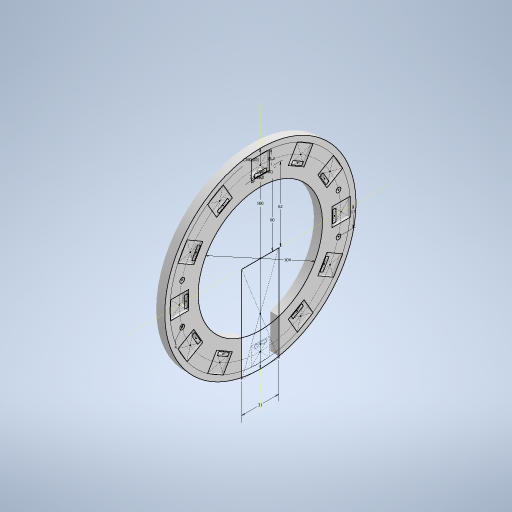
# Autodesk Inventor part: uMule-podstawka_czujnikiIR
Saved by Autodesk Inventor 2024.2 (Build 282272000, 272)
## iProperties
Created: 2024-10-29
Part Number: uMule-podstawka_czujnikiIR
Material: Ogólny
Document SubType Name: Modeling
Designer: owozn
Density: 1 g/cm^3
Appearance: Domyślna
Author: owozn
Autodesk Inventor part; units mm, degrees
ref_plane "YZ Plane" through (0, 0, 0) normal (1, 0, 0) x (0, 1, 0)
ref_plane "XZ Plane" through (0, 0, 0) normal (0, 1, 0) x (-1, 0, 0)
ref_plane "XY Plane" through (0, 0, 0) normal (0, 0, 1) x (1, 0, 0)
sketch "Szkic1" plane through (0, 0, 0) normal (1, 0, 0) x (0, 1, 0)
  line L0 (0, -112) -> (0, 112) construction
  line L1 (-112, 0) -> (112, 0) construction
  circle A0 centre (0, 0) radius 67.6 construction
  line L2 (75.2, 7.6) -> (60, 7.6)
  line L3 (60, 7.6) -> (60, -7.6)
  line L4 (60, -7.6) -> (75.2, -7.6)
  line L5 (75.2, -7.6) -> (75.2, 7.6)
  line L6 (75.2, 7.6) -> (60, -7.6) construction
  line L7 (60, 7.6) -> (75.2, -7.6) construction
  circle A1 centre (0, 0) radius 80
  line L8 (61.3251, 44.1818) -> (48.1615, 36.5818)
  line L9 (48.1615, 36.5818) -> (55.7615, 23.4182)
  line L10 (55.7615, 23.4182) -> (68.9251, 31.0182)
  line L11 (68.9251, 31.0182) -> (61.3251, 44.1818)
  line L12 (61.3251, 44.1818) -> (55.7615, 23.4182) construction
  line L13 (48.1615, 36.5818) -> (68.9251, 31.0182) construction
  line L14 (31.0182, 68.9251) -> (23.4182, 55.7615)
  line L15 (23.4182, 55.7615) -> (36.5818, 48.1615)
  line L16 (36.5818, 48.1615) -> (44.1818, 61.3251)
  line L17 (44.1818, 61.3251) -> (31.0182, 68.9251)
  line L18 (31.0182, 68.9251) -> (36.5818, 48.1615) construction
  line L19 (23.4182, 55.7615) -> (44.1818, 61.3251) construction
  line L20 (-7.6, 75.2) -> (-7.6, 60)
  line L21 (-7.6, 60) -> (7.6, 60)
  line L22 (7.6, 60) -> (7.6, 75.2)
  line L23 (7.6, 75.2) -> (-7.6, 75.2)
  line L24 (-7.6, 75.2) -> (7.6, 60) construction
  line L25 (-7.6, 60) -> (7.6, 75.2) construction
  line L26 (-44.1818, 61.3251) -> (-36.5818, 48.1615)
  line L27 (-36.5818, 48.1615) -> (-23.4182, 55.7615)
  line L28 (-23.4182, 55.7615) -> (-31.0182, 68.9251)
  line L29 (-31.0182, 68.9251) -> (-44.1818, 61.3251)
  line L30 (-44.1818, 61.3251) -> (-23.4182, 55.7615) construction
  line L31 (-36.5818, 48.1615) -> (-31.0182, 68.9251) construction
  line L32 (-68.9251, 31.0182) -> (-55.7615, 23.4182)
  line L33 (-55.7615, 23.4182) -> (-48.1615, 36.5818)
  line L34 (-48.1615, 36.5818) -> (-61.3251, 44.1818)
  line L35 (-61.3251, 44.1818) -> (-68.9251, 31.0182)
  line L36 (-68.9251, 31.0182) -> (-48.1615, 36.5818) construction
  line L37 (-55.7615, 23.4182) -> (-61.3251, 44.1818) construction
  line L38 (-75.2, -7.6) -> (-60, -7.6) construction
  line L39 (-60, -7.6) -> (-60, 7.6) construction
  line L40 (-60, 7.6) -> (-75.2, 7.6) construction
  line L41 (-75.2, 7.6) -> (-75.2, -7.6) construction
  line L42 (-75.2, -7.6) -> (-60, 7.6) construction
  line L43 (-60, -7.6) -> (-75.2, 7.6) construction
  line L44 (-61.3251, -44.1818) -> (-48.1615, -36.5818)
  line L45 (-48.1615, -36.5818) -> (-55.7615, -23.4182)
  line L46 (-55.7615, -23.4182) -> (-68.9251, -31.0182)
  line L47 (-68.9251, -31.0182) -> (-61.3251, -44.1818)
  line L48 (-61.3251, -44.1818) -> (-55.7615, -23.4182) construction
  line L49 (-48.1615, -36.5818) -> (-68.9251, -31.0182) construction
  line L50 (-31.0182, -68.9251) -> (-23.4182, -55.7615)
  line L51 (-23.4182, -55.7615) -> (-36.5818, -48.1615)
  line L52 (-36.5818, -48.1615) -> (-44.1818, -61.3251)
  line L53 (-44.1818, -61.3251) -> (-31.0182, -68.9251)
  line L54 (-31.0182, -68.9251) -> (-36.5818, -48.1615) construction
  line L55 (-23.4182, -55.7615) -> (-44.1818, -61.3251) construction
  line L56 (7.6, -75.2) -> (7.6, -60)
  line L57 (7.6, -60) -> (-7.6, -60)
  line L58 (-7.6, -60) -> (-7.6, -75.2)
  line L59 (-7.6, -75.2) -> (7.6, -75.2)
  line L60 (7.6, -75.2) -> (-7.6, -60) construction
  line L61 (7.6, -60) -> (-7.6, -75.2) construction
  line L62 (44.1818, -61.3251) -> (36.5818, -48.1615)
  line L63 (36.5818, -48.1615) -> (23.4182, -55.7615)
  line L64 (23.4182, -55.7615) -> (31.0182, -68.9251)
  line L65 (31.0182, -68.9251) -> (44.1818, -61.3251)
  line L66 (44.1818, -61.3251) -> (23.4182, -55.7615) construction
  line L67 (36.5818, -48.1615) -> (31.0182, -68.9251) construction
  line L68 (68.9251, -31.0182) -> (55.7615, -23.4182)
  line L69 (55.7615, -23.4182) -> (48.1615, -36.5818)
  line L70 (48.1615, -36.5818) -> (61.3251, -44.1818)
  line L71 (61.3251, -44.1818) -> (68.9251, -31.0182)
  line L72 (68.9251, -31.0182) -> (48.1615, -36.5818) construction
  line L73 (55.7615, -23.4182) -> (61.3251, -44.1818) construction
  line L74 (0, 15.5) -> (-80, 15.5)
  line L75 (-80, 15.5) -> (-80, -15.5) construction
  line L76 (-80, -15.5) -> (0, -15.5)
  line L77 (0, -15.5) -> (0, 15.5)
  line L78 (0, 15.5) -> (-80, -15.5) construction
  line L79 (-80, 15.5) -> (0, -15.5) construction
  circle A2 centre (0, 0) radius 52
  line L80 (63.4, -5) -> (60.6, -5)
  line L81 (60.6, -5) -> (60.6, 5)
  line L82 (60.6, 5) -> (63.4, 5)
  line L83 (63.4, 5) -> (63.4, -5)
  line L84 (63.4, -5) -> (60.6, 5) construction
  line L85 (60.6, -5) -> (63.4, 5) construction
  line L86 (54.9811, 25.9699) -> (49.9811, 34.6301)
  line L87 (49.9811, 34.6301) -> (52.406, 36.0301)
  line L88 (52.406, 36.0301) -> (57.406, 27.3699)
  line L89 (57.406, 27.3699) -> (49.9811, 34.6301) construction
  line L90 (54.9811, 25.9699) -> (52.406, 36.0301) construction
  line L91 (57.406, 27.3699) -> (54.9811, 25.9699)
  line L92 (34.6301, 49.9811) -> (25.9699, 54.9811)
  line L93 (25.9699, 54.9811) -> (27.3699, 57.406)
  line L94 (27.3699, 57.406) -> (36.0301, 52.406)
  line L95 (36.0301, 52.406) -> (25.9699, 54.9811) construction
  line L96 (34.6301, 49.9811) -> (27.3699, 57.406) construction
  line L97 (36.0301, 52.406) -> (34.6301, 49.9811)
  line L98 (5, 60.6) -> (-5, 60.6)
  line L99 (-5, 60.6) -> (-5, 63.4)
  line L100 (-5, 63.4) -> (5, 63.4)
  line L101 (5, 63.4) -> (-5, 60.6) construction
  line L102 (5, 60.6) -> (-5, 63.4) construction
  line L103 (5, 63.4) -> (5, 60.6)
  line L104 (-25.9699, 54.9811) -> (-34.6301, 49.9811)
  line L105 (-34.6301, 49.9811) -> (-36.0301, 52.406)
  line L106 (-36.0301, 52.406) -> (-27.3699, 57.406)
  line L107 (-27.3699, 57.406) -> (-34.6301, 49.9811) construction
  line L108 (-25.9699, 54.9811) -> (-36.0301, 52.406) construction
  line L109 (-27.3699, 57.406) -> (-25.9699, 54.9811)
  line L110 (-49.9811, 34.6301) -> (-54.9811, 25.9699)
  line L111 (-54.9811, 25.9699) -> (-57.406, 27.3699)
  line L112 (-57.406, 27.3699) -> (-52.406, 36.0301)
  line L113 (-52.406, 36.0301) -> (-54.9811, 25.9699) construction
  line L114 (-49.9811, 34.6301) -> (-57.406, 27.3699) construction
  line L115 (-52.406, 36.0301) -> (-49.9811, 34.6301)
  line L116 (-60.6, 5) -> (-60.6, -5) construction
  line L117 (-60.6, -5) -> (-63.4, -5) construction
  line L118 (-63.4, -5) -> (-63.4, 5) construction
  line L119 (-63.4, 5) -> (-60.6, -5) construction
  line L120 (-60.6, 5) -> (-63.4, -5) construction
  line L121 (-63.4, 5) -> (-60.6, 5) construction
  line L122 (-54.9811, -25.9699) -> (-49.9811, -34.6301)
  line L123 (-49.9811, -34.6301) -> (-52.406, -36.0301)
  line L124 (-52.406, -36.0301) -> (-57.406, -27.3699)
  line L125 (-57.406, -27.3699) -> (-49.9811, -34.6301) construction
  line L126 (-54.9811, -25.9699) -> (-52.406, -36.0301) construction
  line L127 (-57.406, -27.3699) -> (-54.9811, -25.9699)
  line L128 (-34.6301, -49.9811) -> (-25.9699, -54.9811)
  line L129 (-25.9699, -54.9811) -> (-27.3699, -57.406)
  line L130 (-27.3699, -57.406) -> (-36.0301, -52.406)
  line L131 (-36.0301, -52.406) -> (-25.9699, -54.9811) construction
  line L132 (-34.6301, -49.9811) -> (-27.3699, -57.406) construction
  line L133 (-36.0301, -52.406) -> (-34.6301, -49.9811)
  line L134 (-5, -60.6) -> (5, -60.6)
  line L135 (5, -60.6) -> (5, -63.4)
  line L136 (5, -63.4) -> (-5, -63.4)
  line L137 (-5, -63.4) -> (5, -60.6) construction
  line L138 (-5, -60.6) -> (5, -63.4) construction
  line L139 (-5, -63.4) -> (-5, -60.6)
  line L140 (25.9699, -54.9811) -> (34.6301, -49.9811)
  line L141 (34.6301, -49.9811) -> (36.0301, -52.406)
  line L142 (36.0301, -52.406) -> (27.3699, -57.406)
  line L143 (27.3699, -57.406) -> (34.6301, -49.9811) construction
  line L144 (25.9699, -54.9811) -> (36.0301, -52.406) construction
  line L145 (27.3699, -57.406) -> (25.9699, -54.9811)
  line L146 (49.9811, -34.6301) -> (54.9811, -25.9699)
  line L147 (54.9811, -25.9699) -> (57.406, -27.3699)
  line L148 (57.406, -27.3699) -> (52.406, -36.0301)
  line L149 (52.406, -36.0301) -> (54.9811, -25.9699) construction
  line L150 (49.9811, -34.6301) -> (57.406, -27.3699) construction
  line L151 (52.406, -36.0301) -> (49.9811, -34.6301)
  circle A3 centre (-17, 65.4275) radius 2
  circle A4 centre (17, 65.4275) radius 2
  circle A5 centre (-17, -65.4275) radius 2
  circle A6 centre (17, -65.4275) radius 2
  point P0 (67.6, 0)
  point P1 (58.5433, 33.8)
  point P2 (33.8, 58.5433)
  point P3 (0, 67.6)
  point P4 (-33.8, 58.5433)
  point P5 (-58.5433, 33.8)
  point P6 (-67.6, 0)
  point P7 (-58.5433, -33.8)
  point P8 (-33.8, -58.5433)
  point P9 (0, -67.6)
  point P10 (33.8, -58.5433)
  point P11 (58.5433, -33.8)
  point P12 (-40, 0)
  point P13 (-49.6362, 15.5)
  point P14 (-49.6362, -15.5)
  point P15 (-78.4841, -15.5)
  point P16 (-78.4841, 15.5)
  point P17 (62, 0)
  point P18 (0, 0)
  point P19 (53.6936, 31)
  point P20 (31, 53.6936)
  point P21 (0, 62)
  point P22 (-31, 53.6936)
  point P23 (-53.6936, 31)
  point P24 (-62, 0)
  point P25 (-53.6936, -31)
  point P26 (-31, -53.6936)
  point P27 (0, -62)
  point P28 (31, -53.6936)
  point P29 (53.6936, -31)
  dimension "d1" = 15.2
  dimension "d2" = 15.2
  dimension "d3" = 160
  dimension "d6" = 360
  dimension "d8" = 60
  dimension "d13" = 31
  dimension "d14" = 104
  dimension "d15" = 2.8
  dimension "d16" = 10
  dimension "d17" = 62
  dimension "d20" = 360
  dimension "d22" = 4
  dimension "d23" = 17
  constraints: 300 end point, 8 midpoint, 7 centre point, 6 parallel, 3 coincident, 3 horizontal, 3 perpendicular, 3 point on line, 3 symmetric about line, 2 point on circle, 1 tangent, 269 other
  measures "d1" distance of L4.end L3.end
  measures "d2" distance of L3.end L2.end
  measures "d3" diameter of A1
  measures "d8" distance from line of point (0, 0) L3
  measures "d13" distance of L75.end L74.end
  measures "d14" diameter of A2
  measures "d15" distance of L81.end L82.end
  measures "d16" distance of L80.end L81.end
  measures "d17" distance of point (0, 0) point (62, 0)
  measures "d22" diameter of A3
  measures "d23" distance from line of L0 A5.centre
extrude "Wyciągnięcie proste1" add sketch "Szkic1" against normal blind 7 contours L5 L4 L3 L2 | A1 L76 A2 L74 | L11 L10 L9 L8 | L17 L16 L15 L14 | L23 L22 L21 L20 | L29 L28 L27 L26 | L35 L34 L33 L32 | L47 L46 L45 L44 | L53 L52 L51 L50 | L59 L58 L57 L56 | L65 L64 L63 L62 | L71 L70 L69 L68 picked at (47.2911, 46.9149)
extrude "Wyciągnięcie proste2" cut sketch "Szkic1" against normal blind 2 contours L5 L4 L3 L2 | L11 L10 L9 L8 | L17 L16 L15 L14 | L23 L22 L21 L20 | L29 L28 L27 L26 | L35 L34 L33 L32 | L47 L46 L45 L44 | L53 L52 L51 L50 | L59 L58 L57 L56 | L65 L64 L63 L62 | L71 L70 L69 L68 | L80 L81 L82 L83 | L86 L87 L88 L91 | L92 L93 L94 L97 | L98 L99 L100 L103 | L104 L105 L106 L109 | L110 L111 L112 L115 | L122 L123 L124 L127 | L128 L129 L130 L133 | L134 L135 L136 L139 | L140 L141 L142 L145 | L146 L147 L148 L151
